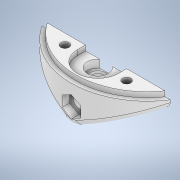
# Autodesk Inventor part: WheelBracketHead
Saved by Autodesk Inventor 2020 (Build 240168000, 168)
## iProperties
Created: 2019-05-28
Part Number: WheelBracketHead
Material: ABS Plastic
Document SubType Name: Modeling
Designer: Connor
Density: 1.06 g/cm^3
Appearance: White
Author: Connor
Autodesk Inventor part; units mm, degrees
ref_plane "YZ Plane" through (0, 0, 0) normal (1, 0, 0) x (0, 1, 0)
sketch "Sketch1" plane through (0, 0, 0) normal (0, 0, 1) x (1, 0, 0)
  line L0 (0, 0) -> (46.99, 0)
  line L1 (46.99, 0) -> (46.99, 22.225)
  line L2 (46.99, 22.225) -> (0, 22.225)
  line L3 (0, 22.225) -> (0, 0)
  line L4 (0, 22.225) -> (44.323, 22.225)
  line L5 (44.323, 22.225) -> (44.323, 25.4254)
  line L6 (44.323, 25.4254) -> (0, 25.4254)
  line L7 (0, 25.4254) -> (0, 22.225)
  circle A0 centre (0, 9.525) radius 9.525
  circle A1 centre (0, 9.525) radius 3.175
  line L8 (46.99, 22.225) -> (4.2364, 0.994)
  line L9 (0, 0) -> (-46.99, 0)
  line L10 (-46.99, 0) -> (-46.99, 22.225)
  line L11 (-46.99, 22.225) -> (0, 22.225)
  line L12 (0, 22.225) -> (0, 0)
  line L13 (-46.99, 22.225) -> (-4.2364, 0.994)
  dimension "d2" = 44.323
  dimension "d3" = 3.2004
  dimension "d5" = 6.35
  dimension "d7" = 6.35
  dimension "d67" = 12.7
  dimension "d119" = 46.99
  constraints: 28 end point, 6 parallel, 3 horizontal, 3 perpendicular, 3 point on circle, 2 centre point, 2 equal length, 2 tangent, 1 coincident, 1 point on line
  measures "d2" distance of L6.end L5.end
  measures "d3" distance of L5.end L4.end
  measures "d5" diameter of A1
  measures "d7" radial gap between concentric circles of A1 A0
  measures "d67" distance from line of L11 A0.centre
  measures "d119" distance between parallel lines of L7 L1
revolve "Revolution1" add sketch "Sketch1" angle 180 about axis through (0, 22.225, 0) along (0, -1, 0) picked at (0.942, 16.8272) picked at (0.9535, 9.9842) contours A0 L8 L1 L0 | L3 A1 A0 | L3 A1 | A0 L3 L2 L8 | L2 L7 L6 L5
sketch "Sketch2" plane through (0, 0, 0) normal (1, 0, 0) x (0, 1, 0)
  line L0 (0, 0) -> (22.225, 0) projected
  line L1 (25.4254, 44.323) -> (25.4254, 0) projected
  line L2 (0, 0) -> (25.4254, 0)
  line L3 (25.4254, 0) -> (25.4254, 25.4)
  line L4 (25.4254, 25.4) -> (0, 25.4)
  line L5 (0, 25.4) -> (0, 0)
  dimension "d10" = 25.4
  constraints: 8 end point, 2 parallel, 1 horizontal, 1 perpendicular, 1 point on line
  measures "d10" distance between parallel lines of L0 L4
extrude "Extrusion1" cut sketch "Sketch2" along normal through all both and the other way through all
extrude "Extrusion2" cut sketch "Sketch1" along normal through all contours A0 L8 L1 L0 | L9 L10 L13 A0
ref_plane "Work Plane1" through (0, 0, 0) normal (0, 1, 0) x (-1, 0, 0)
sketch "Sketch9" plane through (0, 0, 0) normal (0, 1, 0) x (-1, 0, 0)
  line L0 (-19.05, 31.75) -> (0, 0) construction
  line L1 (0, 0) -> (19.05, 31.75) construction
  dimension "d46" = 31.75
  dimension "d47" = 38.1
  constraints: 4 end point, 1 equal length, 1 horizontal alignment
  measures "d46" vertical distance of L0.end L0.start
  measures "d47" distance of L1.end L0.start
hole "Hole1" at (19.05, 0, 31.75) at (-19.05, 0, 31.75) direction (0, 1, 0) diameter 5.207 end through all counterbore diameter 8.7313 counterbore depth 12.7
ref_plane "Work Plane2" through (0, 11.1125, 46.99) normal (0, 0, 1) x (1, 0, 0)
sketch "Sketch10" plane through (0, 11.1125, 46.99) normal (0, 0, 1) x (1, 0, 0)
  arc A0 (-4.2364, -10.1185) -> (4.2364, -10.1185) centre (0, -1.5875) ccw projected
  point P0 (0, -11.1125)
  constraints: 1 coincident
hole "Hole2" at (0, 9.525, 46.99) direction (0, 0, -1) diameter 6.7564 end through all
fillet "Fillet1" radius 0.7937 4 edges at (19.05, 8.3503, 36.1156) (-19.05, 8.3503, 36.1156) (-3.3781, 9.4995, 46.8684) (3.3781, 9.4966, 46.8684)
fillet "Fillet2" radius 3.175 4 edges at (2.2299, 0.2647, 46.9371) (-2.2284, 0.2643, 46.9371) (-24.3604, 10.9873, 40.1825) (24.3604, 10.9873, 40.1825)
sketch "Sketch12" plane through (0, 0, 0) normal (1, 0, 0) x (0, 1, 0)
  line L0 (12.9032, 25.4) -> (6.1468, 25.4) projected
  line L1 (22.225, 17.78) -> (22.225, 30.48)
  line L2 (43.3764, 30.48) -> (22.225, 30.48)
  line L3 (43.3764, 30.48) -> (43.3764, 17.78)
  line L4 (43.3764, 17.78) -> (22.225, 17.78)
  point P0 (0, 0)
  point P1 (9.525, 25.4)
  dimension "d108" = 12.7
  dimension "d111" = 30.48
  dimension "d120" = 12.7
  constraints: 8 end point, 2 vertical, 1 midpoint, 1 perpendicular
  measures "d108" distance from line of point (9.525, 25.4) L1
  measures "d111" distance from line of point (0, 0) L2
  measures "d120" distance between parallel lines of L4 L2
revolve "Revolution2" cut sketch "Sketch12" angle 360 about axis through (0, 43.3764, 30.48) along (0, -1, 0)
sketch "Sketch13" plane through (0, 11.1125, 46.99) normal (0, 0, 1) x (1, 0, 0)
  circle A0 centre (0, -1.5875) radius 3.3782 projected
  line L0 (0, 4.975) -> (5.6832, 1.6937)
  line L1 (5.6832, 1.6937) -> (5.6832, -4.8687)
  line L2 (5.6832, -4.8687) -> (0, -8.15)
  line L3 (0, -8.15) -> (-5.6833, -4.8687)
  line L4 (-5.6833, -4.8687) -> (-5.6832, 1.6937)
  line L5 (-5.6832, 1.6937) -> (0, 4.975)
  point P0 (0, -11.1125)
  dimension "d91" = 11.3665
  constraints: 12 end point, 1 coincident, 1 vertical alignment, 13 other
  measures "d91" distance between parallel lines of L3 L0
extrude "Extrusion8" cut sketch "Sketch13" against normal blind 4.7625
sketch "Sketch14" plane through (39.5335, 22.225, 25.4) normal (0, 0, -1) x (-1, 0, 0)
  line L0 (26.8335, 0) -> (26.8335, 3.2004) projected
  line L1 (52.2335, 0) -> (52.2335, 3.2004) projected
  line L2 (52.2335, 0) -> (26.8335, 0) projected
  line L3 (26.8335, 3.2004) -> (52.2335, 3.2004) projected
  point P0 (39.5335, -22.225)
  point P1 (51.1733, 0)
  point P2 (27.8938, 0)
  point P3 (27.8938, 3.2004)
  point P4 (51.1733, 3.2004)
extrude "Extrusion9" cut sketch "Sketch14" against normal blind 5.08
sketch "Sketch15" plane through (0, 22.225, 30.48) normal (0, 1, 0) x (1, 0, 0)
  circle A0 centre (0, 0) radius 6.477
  arc A1 (-12.7, 0) -> (12.7, 0) centre (0, 0) ccw projected
  point P0 (0, 30.48)
  dimension "d98" = 12.954
  constraints: 1 centre point, 1 coincident, 1 concentric
  measures "d98" diameter of A0
hole "Hole5" at (0, 22.225, 30.48) direction (0, -1, 0) diameter 8.89 depth 6.35 counterbore diameter 12.954 counterbore depth 4.7752
body "Solid1"
